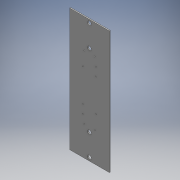
# Autodesk Inventor part: bottom_board
Saved by Autodesk Inventor 2016 (Build 200138000, 138)
## iProperties
Created: 2016-11-05
Part Number: bottom_board
Material: 一般
Document SubType Name: Modeling
Designer: 宏太
Density: 1 g/cm^3
Appearance: 既定
Mass: 41.2921 g
Surface Area: 428.281 cm^2
Volume: 41.2921 cm^3
Author: 宏太
Autodesk Inventor part; units mm, degrees
ref_plane "YZ Plane" through (0, 0, 0) normal (1, 0, 0) x (0, 1, 0)
ref_plane "XZ Plane" through (0, 0, 0) normal (0, 1, 0) x (-1, 0, 0)
ref_plane "XY Plane" through (0, 0, 0) normal (0, 0, 1) x (1, 0, 0)
sketch "スケッチ1" plane through (0, 0, 0) normal (0, 1, 0) x (-1, 0, 0)
  line L0 (0, 0) -> (84, 0)
  line L1 (84, 0) -> (84, -260)
  line L2 (84, -260) -> (0, -260)
  line L3 (0, -260) -> (0, 0)
  dimension "d0" = 84
  dimension "d1" = 260
  constraints: 8 end point, 2 parallel, 1 horizontal, 1 perpendicular
  measures "d0" distance of L1.end L2.end
  measures "d1" distance of L0.end L1.end
extrude "押し出し1" add sketch "スケッチ1" along normal blind 2
sketch "スケッチ2" plane through (0, 0, 0) normal (0, -1, 0) x (1, 0, 0)
  circle A0 centre (-42, -7) radius 4
  line L0 (0, -260) -> (0, 0) projected
  line L1 (0, 0) -> (-84, 0) projected
  circle A1 centre (-42, -53) radius 4
  circle A2 centre (-42, -253) radius 4
  circle A3 centre (-42, -207) radius 4
  line L2 (-84, -260) -> (0, -260) projected
  circle A4 centre (-28.5, -80) radius 1
  circle A5 centre (-28.5, -98) radius 1
  circle A6 centre (-55.5, -93) radius 1
  circle A7 centre (-53, -62.5) radius 1
  circle A8 centre (-31, -62.5) radius 1
  circle A9 centre (-31, -197.5) radius 1
  circle A10 centre (-53, -197.5) radius 1
  circle A11 centre (-55.5, -180) radius 1
  circle A12 centre (-55.5, -162) radius 1
  circle A13 centre (-28.5, -167) radius 1
  dimension "d4" = 8
  dimension "d6" = 42
  dimension "d7" = 7
  dimension "d8" = 8
  dimension "d10" = 42
  dimension "d11" = 8
  dimension "d12" = 8
  dimension "d13" = 42
  dimension "d14" = 7
  dimension "d15" = 42
  dimension "d29" = 46
  dimension "d30" = 2
  dimension "d32" = 80
  dimension "d33" = 2
  dimension "d35" = 2
  dimension "d37" = 93
  dimension "d38" = 53
  dimension "d39" = 55.5
  dimension "d40" = 28.5
  dimension "d41" = 28.5
  dimension "d42" = 2
  dimension "d44" = 62.5
  dimension "d45" = 2
  dimension "d47" = 62.5
  dimension "d48" = 53
  dimension "d49" = 31
  dimension "d57" = 98
  dimension "d58" = 2
  dimension "d59" = 31
  dimension "d60" = 197.5
  dimension "d61" = 2
  dimension "d62" = 53
  dimension "d63" = 197.5
  dimension "d64" = 2
  dimension "d65" = 55.5
  dimension "d66" = 180
  dimension "d67" = 2
  dimension "d68" = 55.5
  dimension "d69" = 162
  dimension "d70" = 2
  dimension "d71" = 28.5
  dimension "d72" = 167
  constraints: 14 centre point
  measures "d4" diameter of A0
  measures "d6" distance from line of L0 A0.centre
  measures "d7" distance from line of L1 A0.centre
  measures "d8" diameter of A1
  measures "d10" distance from line of L0 A1.centre
  measures "d11" diameter of A2
  measures "d12" diameter of A3
  measures "d13" distance from line of L0 A2.centre
  measures "d14" distance from line of L2 A2.centre
  measures "d15" distance from line of L0 A3.centre
  measures "d29" distance of A2.centre A3.centre
  measures "d30" diameter of A4
  measures "d32" distance from line of L1 A4.centre
  measures "d33" diameter of A5
  measures "d35" diameter of A6
  measures "d37" distance from line of L1 A6.centre
  measures "d38" distance from line of L1 A1.centre
  measures "d39" distance from line of L0 A6.centre
  measures "d40" distance from line of L0 A5.centre
  measures "d41" distance from line of L0 A4.centre
  measures "d42" diameter of A7
  measures "d44" distance from line of L1 A7.centre
  measures "d45" diameter of A8
  measures "d47" distance from line of L1 A8.centre
  measures "d48" distance from line of L0 A7.centre
  measures "d49" distance from line of L0 A8.centre
  measures "d57" distance from line of L1 A5.centre
  measures "d58" diameter of A9
  measures "d59" distance from line of L0 A9.centre
  measures "d60" distance from line of L1 A9.centre
  measures "d61" diameter of A10
  measures "d62" distance from line of L0 A10.centre
  measures "d63" distance from line of L1 A10.centre
  measures "d64" diameter of A11
  measures "d65" distance from line of L0 A11.centre
  measures "d66" distance from line of L1 A11.centre
  measures "d67" diameter of A12
  measures "d68" distance from line of L0 A12.centre
  measures "d69" distance from line of L1 A12.centre
  measures "d70" diameter of A13
  measures "d71" distance from line of L0 A13.centre
  measures "d72" distance from line of L1 A13.centre
extrude "押し出し6" cut sketch "スケッチ2" against normal blind 2
